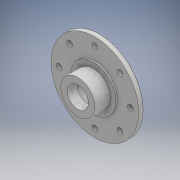
# Autodesk Inventor part: Lower Cylinder Cover
Saved by Autodesk Inventor 2017 (Build 210142000, 142)
## iProperties
Created: 2018-11-17
Part Number: Lower Cylinder Cover
Material: Generic
Document SubType Name: Modeling
Designer: Arman Grewal
Density: 1 g/cm^3
Appearance: Default
Author: Arman Grewal
Autodesk Inventor part; units mm, degrees
ref_plane "YZ Plane" through (0, 0, 0) normal (1, 0, 0) x (0, 1, 0)
ref_plane "XZ Plane" through (0, 0, 0) normal (0, 1, 0) x (-1, 0, 0)
ref_plane "XY Plane" through (0, 0, 0) normal (0, 0, 1) x (1, 0, 0)
sketch "Sketch1" plane through (0, 0, 0) normal (0, 1, 0) x (-1, 0, 0)
  circle A0 centre (0, 0) radius 27
  dimension "d0" = 54
  constraints: 1 centre point, 1 coincident
  measures "d0" diameter of A0
extrude "Extrusion1" add sketch "Sketch1" along normal blind 3
sketch "Sketch2" plane through (0, 3, 0) normal (0, 1, 0) x (1, 0, 0)
  circle A0 centre (0, 0) radius 16
  dimension "d4" = 32
  constraints: 1 centre point, 1 coincident
  measures "d4" diameter of A0
extrude "Extrusion2" add sketch "Sketch2" along normal blind 1.5
sketch "Sketch3" plane through (0, 0, 0) normal (0, -1, 0) x (1, 0, 0)
  circle A0 centre (0, 0) radius 14
  dimension "d7" = 28
  constraints: 1 centre point, 1 coincident
  measures "d7" diameter of A0
extrude "Extrusion3" add sketch "Sketch3" along normal blind 1
sketch "Sketch4" plane through (0, -1, 0) normal (0, -1, 0) x (1, 0, 0)
  circle A0 centre (0, 0) radius 10.5
  dimension "d10" = 21
  constraints: 1 centre point, 1 coincident
  measures "d10" diameter of A0
extrude "Extrusion4" add sketch "Sketch4" along normal blind 9.5
sketch "Sketch6" plane through (0, 4.5, 0) normal (0, 1, 0) x (1, 0, 0)
  circle A0 centre (0, 0) radius 3
  dimension "d14" = 6
  constraints: 1 centre point, 1 coincident
  measures "d14" diameter of A0
extrude "Extrusion5" cut sketch "Sketch6" against normal through all
sketch "Sketch7" plane through (0, 3, 0) normal (0, 1, 0) x (1, 0, 0)
  circle A0 centre (0, 0) radius 22 construction
  circle A1 centre (0, 22) radius 1.75
  circle A2 centre (-15.5563, 15.5563) radius 1.75
  circle A3 centre (-22, 0) radius 1.75
  circle A4 centre (-15.5563, -15.5563) radius 1.75
  circle A5 centre (0, -22) radius 1.75
  circle A6 centre (15.5563, -15.5563) radius 1.75
  circle A7 centre (22, 0) radius 1.75
  circle A8 centre (15.5563, 15.5563) radius 1.75
  dimension "d17" = 44
  dimension "d18" = 3.5
  dimension "d21" = 360
  dimension "d23" = 6.4436
  constraints: 8 centre point, 1 coincident, 1 vertical alignment, 19 other
  measures "d18" diameter of A1
  measures "d23" vertical distance of A8.centre A1.centre
extrude "Extrusion6" cut sketch "Sketch7" against normal blind 3
sketch "Sketch9" plane through (0, -10.5, 0) normal (0, -1, 0) x (1, 0, 0)
  circle A0 centre (0, 0) radius 6.5
  dimension "d26" = 13
  constraints: 1 centre point, 1 coincident
  measures "d26" diameter of A0
extrude "Extrusion7" cut sketch "Sketch9" against normal blind 9.5
chamfer "Chamfer1" distance 3.5 angle 45 1 edges at (-6.5, -1, 0)
fillet "Fillet1" radius 0.25 1 edges at (27, 3, 0)
body "Solid1"
